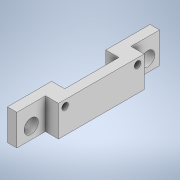
# Autodesk Inventor part: arduino_clamp
Saved by Autodesk Inventor 2022 (Build 260153000, 153)
## iProperties
Created: 2022-01-21
Part Number: arduino_clamp
Material: Generic
Document SubType Name: Modeling
Designer: kylem
Density: 1 g/cm^3
Appearance: Default
Author: kylem
Autodesk Inventor part; units mm, degrees
ref_plane "YZ Plane" through (0, 0, 0) normal (1, 0, 0) x (0, 1, 0)
ref_plane "XZ Plane" through (0, 0, 0) normal (0, 1, 0) x (-1, 0, 0)
ref_plane "XY Plane" through (0, 0, 0) normal (0, 0, 1) x (1, 0, 0)
sketch "Sketch1" plane through (0, 0, 0) normal (1, 0, 0) x (0, 1, 0)
  line L0 (0, 0) -> (6.5, 0)
  line L1 (6.5, 0) -> (6.5, -18)
  line L2 (6.5, -18) -> (0, -18)
  line L3 (0, -18) -> (0, 0)
  dimension "d0" = 6.5
  dimension "d1" = 18
  constraints: 8 end point, 2 parallel, 1 horizontal, 1 perpendicular
  measures "d0" distance of L1.end L2.end
  measures "d1" distance of L0.end L1.end
extrude "Extrusion1" add sketch "Sketch1" along normal blind 2.75
sketch "Sketch2" plane through (2.75, 0, 0) normal (1, 0, 0) x (0, 0, -1)
  line L0 (0, 6.5) -> (0, 0) projected
  line L1 (0, 0) -> (18, 0) projected
  line L2 (0, 6.5) -> (3.3, 6.5)
  line L3 (3.3, 6.5) -> (3.3, 0)
  line L4 (3.3, 0) -> (0, 0)
  line L5 (0, 0) -> (0, 6.5)
  line L6 (18, 0) -> (18, 6.5) projected
  line L7 (18, 6.5) -> (0, 6.5) projected
  line L8 (18, 0) -> (14.7, 0)
  line L9 (14.7, 0) -> (14.7, 6.5)
  line L10 (14.7, 6.5) -> (18, 6.5)
  line L11 (18, 6.5) -> (18, 0)
  line L12 (3.3, 6.5) -> (14.7, 6.5)
  line L13 (14.7, 6.5) -> (14.7, 0)
  line L14 (14.7, 0) -> (3.3, 0)
  line L15 (3.3, 0) -> (3.3, 6.5)
  dimension "d4" = 3.3
  dimension "d5" = 3.3
  constraints: 24 end point, 6 parallel, 3 horizontal, 3 perpendicular, 2 point on line
  measures "d4" distance of L3.end L4.end
  measures "d5" distance of L9.end L10.end
extrude "Extrusion2" cut sketch "Sketch2" against normal blind 2.75 contours L7 L9 L1 L3
sketch "Sketch3" plane through (2.75, 0, 0) normal (1, 0, 0) x (0, 0, -1)
  line L0 (18, 6.5) -> (14.7, 6.5) projected
  line L1 (0, 0) -> (18, 0)
  line L2 (18, 0) -> (18, 6.5)
  line L3 (18, 6.5) -> (0, 6.5)
  line L4 (0, 6.5) -> (0, 0)
  constraints: 8 end point, 2 parallel, 1 horizontal, 1 perpendicular
extrude "Extrusion3" add sketch "Sketch3" along normal blind 2
sketch "Sketch4" plane through (4.75, 0, 0) normal (1, 0, 0) x (0, 0, -1)
  line L0 (3.3, 6.5) -> (0, 6.5) projected
  line L1 (0, 6.5) -> (1.38, 6.5)
  line L2 (1.38, 6.5) -> (1.38, 5.26)
  line L3 (18, 6.5) -> (14.7, 6.5) projected
  line L4 (18, 6.5) -> (16.62, 6.5)
  line L5 (16.62, 6.5) -> (16.62, 5.26)
  circle A0 centre (1.38, 5.26) radius 0.7
  circle A1 centre (16.62, 5.26) radius 0.7
  point P0 (0, 0)
  dimension "d10" = 1.38
  dimension "d11" = 1.24
  dimension "d12" = 1.38
  dimension "d13" = 1.24
  dimension "d14" = 1.4
  dimension "d15" = 1.4
  constraints: 8 end point, 2 centre point, 2 coincident, 2 perpendicular, 2 point on line
  measures "d10" distance of L0.end L1.end
  measures "d11" distance of L1.end L2.end
  measures "d12" distance of L3.start L4.end
  measures "d13" distance of L4.end L5.end
  measures "d14" diameter of A0
  measures "d15" diameter of A1
extrude "Extrusion4" cut sketch "Sketch4" against normal blind 20
sketch "Sketch5" plane through (0, 0, 0) normal (-1, 0, 0) x (0, 0, 1)
  line L0 (-18, 6.5) -> (0, 6.5) projected
  line L1 (0, 6.5) -> (6, 6.5)
  line L2 (6, 6.5) -> (6, 0)
  line L3 (6, 0) -> (0, 0)
  line L4 (0, 0) -> (0, 6.5)
  line L5 (-18, 0) -> (-18, 6.5) projected
  line L6 (-18, 6.5) -> (-24, 6.5)
  line L7 (-24, 6.5) -> (-24, 0)
  line L8 (-24, 0) -> (-18, 0)
  line L9 (-18, 0) -> (-18, 6.5)
  line L10 (-24, 3.25) -> (-21.5, 3.25)
  line L11 (-24, 6.5) -> (-24, 2.5)
  line L12 (-24, 2.5) -> (-21.5, 2.5)
  circle A0 centre (-21.5, 2.5) radius 1.5
  line L13 (6, 6.5) -> (6, 2.5)
  line L14 (6, 2.5) -> (3, 2.5)
  circle A1 centre (3, 2.5) radius 1.5
  point P0 (0, 0)
  dimension "d18" = 6
  dimension "d19" = 6.5
  dimension "d20" = 6
  dimension "d21" = 6.5
  dimension "d27" = 2.5
  dimension "d28" = 4
  dimension "d29" = 2.5
  dimension "d30" = 3
  dimension "d31" = 4
  dimension "d32" = 3
  dimension "d33" = 3
  constraints: 26 end point, 4 perpendicular, 3 horizontal, 3 parallel, 2 centre point, 2 coincident, 2 point on line, 1 midpoint
  measures "d18" distance of L2.end L3.end
  measures "d19" distance of L1.end L2.end
  measures "d20" distance of L8.end L7.end
  measures "d21" distance of L7.end L6.end
  measures "d27" distance of L10.start L10.end
  measures "d28" distance of L6.end L11.end
  measures "d29" distance of L11.end L12.end
  measures "d30" diameter of A0
  measures "d31" distance of L1.end L13.end
  measures "d32" distance of L13.end L14.end
  measures "d33" diameter of A1
extrude "Extrusion6" add sketch "Sketch5" against normal blind 2 contours L1 L2 L3 L4 | L5 L8 L7 L12 A0 L10 L6 | L10 A0 L12 L7
body "Solid1"
